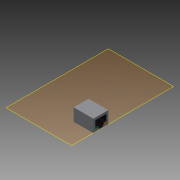
# Autodesk Inventor part: nanopc_t4_rj45
Saved by Autodesk Inventor 2013 SP2 (Build 170200200, 200)
## iProperties
Created: 2018-09-03
Part Number: nanopc_t4_rj45
Material: Generic
Document SubType Name: Modeling
Designer: alex
Density: 1 g/cm^3
Mass: 3.43949 g
Surface Area: 21.8258 cm^2
Volume: 3.43949 cm^3
Author: alex
Autodesk Inventor part; units mm, degrees
ref_plane "YZ Plane" through (0, 0, 0) normal (1, 0, 0) x (0, 1, 0)
ref_plane "XZ Plane" through (0, 0, 0) normal (0, 1, 0) x (-1, 0, 0)
ref_plane "XY Plane" through (0, 0, 0) normal (0, 0, 1) x (1, 0, 0)
ref_plane "Work Plane1" through (0, 0, 0) normal (0, 0, 1) x (1, 0, 0)
sketch "Sketch1" plane through (0, 0, 0) normal (0, 0, 1) x (1, 0, 0)
  line L0 (14.1799, -15.6518) -> (35.3799, -15.6518)
  line L1 (35.3799, -15.6518) -> (35.3799, -31.6518)
  line L2 (35.3799, -31.6518) -> (14.1799, -31.6518)
  line L3 (14.1799, -31.6518) -> (14.1799, -15.6518)
  point P0 (0, 0)
  dimension "d0" = 21.2
  dimension "d2" = 16
  constraints: 8 end point, 2 parallel, 1 horizontal, 1 perpendicular
  measures "d0" distance of L1.end L2.end
  measures "d2" distance of L2.end L0.start
extrude "Extrusion1" add sketch "Sketch1" along normal blind 13.4
sketch "Sketch2" plane through (35.3799, -31.6518, 0) normal (1, 0, 0) x (0, 0, -1)
  line L0 (0, 16) -> (0, 0) projected
  line L1 (0, 16) -> (-13.4, 16) projected
  line L2 (-13.4, 0) -> (-13.4, 16) projected
  line L3 (0, 0) -> (-13.4, 0) projected
  line L4 (-10.9, 2) -> (-4.3, 2)
  line L5 (-4.3, 2) -> (-4.3, 5)
  line L6 (-4.3, 5) -> (-2.5, 5)
  line L7 (-2.5, 5) -> (-2.5, 6)
  line L8 (-2.5, 6) -> (-1, 6)
  line L9 (-1, 6) -> (-1, 10)
  line L10 (-1, 10) -> (-2.5, 10)
  line L11 (-2.5, 10) -> (-2.5, 11)
  line L12 (-2.5, 11) -> (-4.3, 11)
  line L13 (-4.3, 11) -> (-4.3, 14)
  line L14 (-4.3, 14) -> (-10.9, 14)
  line L15 (-10.9, 14) -> (-10.9, 2)
  point P0 (0, 31.6518)
  dimension "d5" = 2
  dimension "d6" = 2
  dimension "d7" = 2.5
  dimension "d8" = 5
  dimension "d9" = 6
  dimension "d10" = 1
  dimension "d11" = 2.5
  dimension "d12" = 4.3
  constraints: 24 end point, 10 parallel, 4 equal length, 1 collinear, 1 perpendicular
  measures "d5" distance between parallel lines of L3 L4
  measures "d6" distance between parallel lines of L1 L14
  measures "d7" distance between parallel lines of L2 L15
  measures "d8" distance between parallel lines of L1 L12
  measures "d9" distance between parallel lines of L1 L10
  measures "d10" distance between parallel lines of L0 L9
  measures "d11" distance between parallel lines of L0 L7
  measures "d12" distance between parallel lines of L0 L5
extrude "Extrusion2" cut sketch "Sketch2" against normal blind 11.5 contours L15 L14 L13 L12 L11 L10 L9 L8 L7 L6 L5 L4
sketch "Sketch3" plane through (35.3799, -31.6518, 0) normal (1, 0, 0) x (0, 0, -1)
  line L0 (-4.3, 5) -> (-4.3, 2) projected
  line L1 (-4.3, 2) -> (-10.9, 2) projected
  line L2 (-10.9, 14) -> (-4.3, 14) projected
  line L3 (-4.3, 14) -> (-4.3, 11) projected
  line L4 (-4.3, 11) -> (-2.5, 11) projected
  line L5 (-2.5, 5) -> (-4.3, 5) projected
  line L6 (-4.1, 4.8) -> (-2.5, 4.8)
  line L7 (-2.5, 4.8) -> (-2.5, 2)
  line L8 (-2.5, 2) -> (-4.1, 2)
  line L9 (-4.1, 2) -> (-4.1, 4.8)
  line L10 (-4.1, 11.2) -> (-2.5, 11.2)
  line L11 (-2.5, 11.2) -> (-2.5, 14)
  line L12 (-2.5, 14) -> (-4.1, 14)
  line L13 (-4.1, 14) -> (-4.1, 11.2)
  point P0 (0, 31.6518)
  dimension "d15" = 0.2
  dimension "d16" = 0.2
  dimension "d17" = 0.2
  dimension "d18" = 0.2
  constraints: 16 end point, 4 parallel, 2 horizontal, 2 perpendicular, 2 point on line
  measures "d15" distance between parallel lines of L6 L5
  measures "d16" distance between parallel lines of L0 L9
  measures "d17" distance between parallel lines of L4 L10
  measures "d18" distance between parallel lines of L3 L13
extrude "Extrusion3" cut sketch "Sketch3" against normal blind 0.2
body "Solid1"
